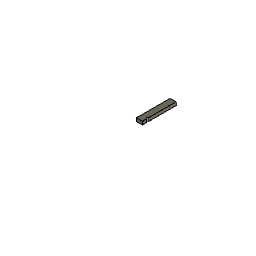
pms bracket (Autodesk Fusion 360 design; units mm, degrees)
Autodesk Fusion 360 part; units mm, degrees
ref_plane "WorkPlane1" through (8, 31, -21.5) normal (0, 0, 1) x (1, 0, 0)
sketch "Sketch1" plane through (8, 31, -21.5) normal (0, 0, 1) x (1, 0, 0)
  line L0 (2.8723, 29.3965) -> (-2.8723, 29.3965)
  line L1 (-2.8723, 29.3965) -> (-2.8723, -2.6479)
  line L2 (-2.8723, -2.6479) -> (2.8723, -2.6479)
  line L3 (2.8723, -2.6479) -> (2.8723, 29.3965)
  constraint horizontal L0
  constraint vertical L1
  constraint horizontal L2
  constraint vertical L3
extrude "Extrude1" add sketch "Sketch1" along normal blind 3
sketch "Sketch2" plane through (0, 0, -18.5) normal (0, 0, 1) x (-1, 0, 0)
  line L0 (-10.8723, -28.3521) -> (-10.8723, -60.3965)
  line L1 (-10.8723, -60.3965) -> (-5.1277, -60.3965)
  line L2 (-5.1277, -60.3965) -> (-5.1277, -28.3521)
  line L3 (-5.1277, -28.3521) -> (-10.8723, -28.3521)
  circle A0 centre (-11, -7) radius 1.2
  circle A1 centre (-11.0423, -33.3352) radius 1.2
  dimension "d79" = 2.4
  dimension "d81" = 2.4
  measures "d79" diameter of A0
  measures "d81" diameter of A1
extrude "Extrude2" cut sketch "Sketch2" against normal blind 11 contours L0 A1 | L0 A1 | A0
